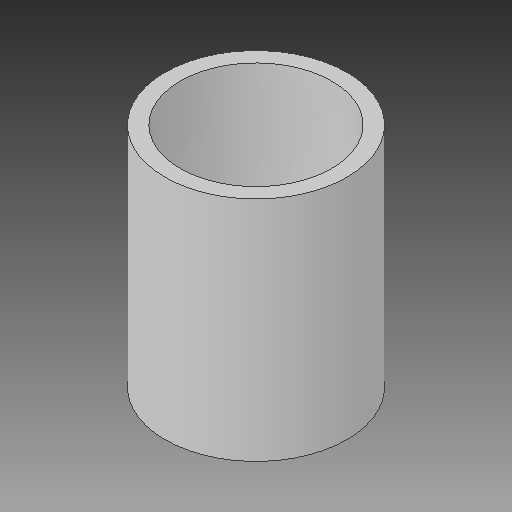
# Autodesk Inventor part: Rodamiento
Saved by Autodesk Inventor 2017 (Build 210142000, 142)
## iProperties
Part Number: Rodamiento
Material: Genérico
Document SubType Name: Modeling
Designer: osvaldo
Density: 1 g/cm^3
Appearance: Valor por defecto
Author: osvaldo
Autodesk Inventor part; units mm, degrees
ref_plane "YZ Plane" through (0, 0, 0) normal (1, 0, 0) x (0, 1, 0)
ref_plane "XZ Plane" through (0, 0, 0) normal (0, 1, 0) x (-1, 0, 0)
ref_plane "XY Plane" through (0, 0, 0) normal (0, 0, 1) x (1, 0, 0)
sketch "Boceto1" plane through (0, 0, 0) normal (0, 1, 0) x (-1, 0, 0)
  circle A0 centre (0, 0) radius 5
  circle A1 centre (0, 0) radius 6
  dimension "d0" = 10
  dimension "d1" = 1
  constraints: 2 centre point, 1 coincident
  measures "d0" diameter of A0
  measures "d1" radial gap between concentric circles of A0 A1
extrude "Extrusión1" add sketch "Boceto1" along normal blind 15
equation "\"d0\" = 10 * scale"
equation "\"d1\" = scale"
equation "\"d2\" = 15 * scale"
equation "\"scale\" = 1"
